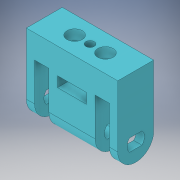
# Autodesk Inventor part: joint1_level
Saved by Autodesk Inventor 2019 (Build 230136000, 136)
## iProperties
Created: 2019-12-26
Part Number: joint1_level
Material: Пластик АБС
Document SubType Name: Modeling
Designer: Петров Иван
Density: 1.06 g/cm^3
Appearance: Серо-синий
Author: Петров Иван
Autodesk Inventor part; units mm, degrees
ref_plane "YZ Plane" through (0, 0, 0) normal (1, 0, 0) x (0, 1, 0)
ref_plane "XZ Plane" through (0, 0, 0) normal (0, 1, 0) x (-1, 0, 0)
sketch "Эскиз1" plane through (0, 0, 0) normal (1, 0, 0) x (0, 1, 0)
  line L0 (-6, -6.0208) -> (-6, 6.0208)
  arc A0 (-6, -6.0208) -> (6, -6.0208) centre (0, 0) ccw
  line L1 (6, 6.0208) -> (6, -6.0208)
  arc A1 (6, 6.0208) -> (-6, 6.0208) centre (0, 0) ccw
  circle A2 centre (0, 0) radius 17.5
  line L2 (0, 17.5) -> (60, 17.5)
  line L3 (60, 17.5) -> (60, -17.5)
  line L4 (60, -17.5) -> (0, -17.5)
  line L5 (0, -17.5) -> (0, -8.5)
  line L6 (0, 8.5) -> (0, 17.5)
  dimension "d0" = 35
  dimension "d1" = 60
  constraints: 14 end point, 6 point on circle, 3 parallel, 2 centre point, 1 coincident, 1 horizontal, 1 perpendicular, 1 vertical alignment, 2 other
  measures "d1" distance of L3.end L4.end
extrude "Выдавливание1" add sketch "Эскиз1" along normal blind 45 contours A0 L5 A2 L6 A1 L0 | A0 L1 A1 L6 A2 L5 | A2 L2 L3 L4
sketch "Эскиз2" plane through (45, 0, 0) normal (1, 0, 0) x (0, 0, -1)
  line L0 (17.5, 60) -> (-17.5, 60) projected
  line L1 (17.5, 0) -> (17.5, 60) projected
  line L2 (-17.5, 60) -> (17.5, 60)
  line L3 (17.5, 60) -> (17.5, 37)
  line L4 (17.5, 37) -> (-17.5, 37)
  line L5 (-17.5, 37) -> (-17.5, 60)
  point P0 (0, 0)
  dimension "d4" = 23
  constraints: 8 end point, 2 parallel, 1 horizontal, 1 perpendicular, 1 point on line
  measures "d4" distance of L2.end L3.end
extrude "Выдавливание2" add sketch "Эскиз2" along normal blind 22
ref_plane "РабПлоскость1" through (22.5, 0, 17.5) normal (1, 0, 0) x (0, 0, -1)
mirror "Зеркальное отражение1" about plane through (22.5, 0, 17.5) normal (1, 0, 0) of "Выдавливание2"
sketch "Эскиз3" plane through (45, 0, 0) normal (1, 0, 0) x (0, 0, -1)
  arc A0 (6.0208, -6) -> (6.0208, 6) centre (0, 0) ccw projected
  line L0 (6.0208, -6) -> (-6.0208, -6) projected
  arc A1 (-6.0208, 6) -> (-6.0208, -6) centre (0, 0) ccw projected
  line L1 (6.0208, 6) -> (-6.0208, 6) projected
  line L2 (17.5, 37) -> (-17.5, 37) projected
  line L3 (-17.5, 37) -> (-17.5, 0) projected
  arc A2 (-17.5, 0) -> (17.5, 0) centre (0, 0) ccw projected
  line L4 (17.5, 0) -> (17.5, 37) projected
sketch "Эскиз4" plane through (67, 0, 0) normal (1, 0, 0) x (0, 0, -1)
  arc A0 (6.0208, -6) -> (6.0208, 6) centre (0, 0) ccw
  line L0 (6.0208, -6) -> (-6.0208, -6)
  arc A1 (-6.0208, 6) -> (-6.0208, -6) centre (0, 0) ccw
  line L1 (6.0208, 6) -> (-6.0208, 6)
  line L2 (17.5, 37) -> (-17.5, 37)
  line L3 (-17.5, 37) -> (-17.5, 0)
  arc A2 (-17.5, 0) -> (17.5, 0) centre (0, 0) ccw
  line L4 (17.5, 0) -> (17.5, 37)
  constraints: 10 end point, 6 point on circle, 3 centre point
extrude "Выдавливание3" add sketch "Эскиз4" against normal blind 8
mirror "Зеркальное отражение2" about plane through (22.5, 0, 17.5) normal (1, 0, 0) of "Выдавливание3"
sketch "Эскиз5" plane through (67, 60, 17.5) normal (0, 1, 0) x (1, 0, 0)
  line L0 (-89, 35) -> (-89, 0) projected
  line L1 (-89, 35.1034) -> (-89, 0)
  line L2 (-89, 0) -> (-89, 35.1034)
  line L3 (-89, 35) -> (0, 35) projected
  line L4 (-89, 35) -> (0, 35)
  line L5 (-89, 17.5517) -> (-44.5, 17.5517)
  circle A0 centre (-44.5, 17.5517) radius 4.1
  line L6 (-44.5, 17.5517) -> (-59.5, 17.5517)
  circle A1 centre (-59.5, 17.5517) radius 7.5
  line L7 (-44.5, 17.5517) -> (-29.5, 17.5517)
  circle A2 centre (-29.5, 17.5517) radius 7.5
  point P0 (-67, 17.5)
  dimension "d9" = 8.2
  dimension "d10" = 15
  dimension "d11" = 15
  dimension "d12" = 15
  dimension "d13" = 15
  constraints: 12 end point, 3 centre point, 3 coincident, 3 collinear, 2 horizontal, 1 midpoint, 1 point on line
  measures "d9" diameter of A0
  measures "d10" distance of L6.start L6.end
  measures "d11" diameter of A1
  measures "d12" distance of L6.start L7.end
  measures "d13" diameter of A2
extrude "Выдавливание4" cut sketch "Эскиз5" against normal blind 10 contours L5 A1 | L5 A1 | A2
sketch "Эскиз6" plane through (67, 60, 17.5) normal (0, 1, 0) x (1, 0, 0)
  line L0 (-89, 35) -> (-89, 0)
  line L1 (-89, 35.1034) -> (-89, 0)
  line L2 (-89, 0) -> (-89, 35.1034)
  line L3 (-89, 35) -> (0, 35)
  line L4 (-89, 35) -> (0, 35)
  line L5 (-89, 17.5517) -> (-44.5, 17.5517)
  circle A0 centre (-44.5, 17.5517) radius 4.1
  line L6 (-44.5, 17.5517) -> (-59.5, 17.5517)
  circle A1 centre (-59.5, 17.5517) radius 7.5
  line L7 (-44.5, 17.5517) -> (-29.5, 17.5517)
  circle A2 centre (-29.5, 17.5517) radius 7.5
  point P0 (-67, 17.5)
  point P1 (-67, 17.5)
  dimension "d16" = 8.2
  dimension "d17" = 15
  dimension "d18" = 15
  dimension "d19" = 15
  dimension "d20" = 15
  constraints: 16 end point, 3 centre point, 3 coincident, 3 collinear, 2 horizontal, 1 midpoint, 1 point on line
  measures "d16" diameter of A0
  measures "d17" distance of L6.start L6.end
  measures "d18" diameter of A1
  measures "d19" distance of L6.start L7.end
  measures "d20" diameter of A2
extrude "Выдавливание5" cut sketch "Эскиз6" against normal blind 35 contours A0 L7 L5 | L5 L7 A0
sketch "Эскиз7" plane through (0, 0, 17.5) normal (0, 0, 1) x (1, 0, 0)
  line L0 (18.4, 60) -> (18.4, 25) projected
  line L1 (26.6, 60) -> (26.6, 25) projected
  line L2 (0, 37) -> (0, 0) projected
  line L3 (45, 0) -> (0, 0) projected
  line L4 (45, 37) -> (45, 0) projected
  line L5 (45, 37) -> (59, 37) projected
  line L6 (59, 0) -> (59, 37) projected
  line L7 (67, 0) -> (59, 0) projected
  line L8 (67, 60) -> (67, 0) projected
  line L9 (-22, 60) -> (67, 60) projected
  line L10 (-22, 60) -> (-22, 0) projected
  line L11 (-22, 0) -> (-14, 0) projected
  line L12 (-14, 0) -> (-14, 37) projected
  line L13 (0, 37) -> (-14, 37) projected
  line L14 (18.4, 25) -> (26.6, 25) projected
  line L15 (18.4, 25) -> (8.4, 25)
  line L16 (8.4, 25) -> (8.4, 35)
  line L17 (8.4, 35) -> (36.6, 35)
  line L18 (36.6, 35) -> (36.6, 25)
  line L19 (26.6, 25) -> (36.6, 25)
  line L20 (18.4, 25) -> (26.6, 25)
  dimension "d23" = 10
  dimension "d24" = 10
  dimension "d25" = 28.2
  dimension "d26" = 10
  constraints: 12 end point, 4 perpendicular, 1 collinear, 1 horizontal, 1 point on line
  measures "d23" distance of L0.end L15.end
  measures "d24" distance of L15.end L16.end
  measures "d25" distance of L16.end L17.end
  measures "d26" distance of L1.end L18.end
extrude "Выдавливание6" cut sketch "Эскиз7" against normal blind 84.5 contours L17 L1 L14 L0 | L0 L15 L16 L17 | L17 L18 L19 L1
